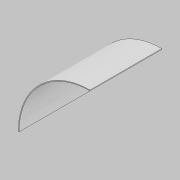
# Autodesk Inventor part: cover2_shell_large
Saved by Autodesk Inventor 2021 (Build 250183000, 183)
## iProperties
Created: 2021-05-31
Part Number: cover2_shell_large
Material: Generic
Document SubType Name: Modeling
Designer: Watchdog
Density: 1 g/cm^3
Appearance: Default
Author: Watchdog
Autodesk Inventor part; units mm, degrees
ref_plane "YZ Plane" through (0, 0, 0) normal (1, 0, 0) x (0, 1, 0)
ref_plane "XZ Plane" through (0, 0, 0) normal (0, 1, 0) x (-1, 0, 0)
ref_plane "XY Plane" through (0, 0, 0) normal (0, 0, 1) x (1, 0, 0)
sketch "Sketch1" plane through (0, 0, 0) normal (0, 0, 1) x (1, 0, 0)
  arc A0 (0, 900) -> (-900, 0) centre (0, 0) ccw
  arc A1 (0, 890) -> (-890, 0) centre (0, 0) ccw
  line L0 (-900, 0) -> (-890, 0)
  line L1 (0, 900) -> (0, 890)
  dimension "d0" = 10
  dimension "d1" = 900
  dimension "d2" = 0
  dimension "d3" = 0
  constraints: 4 end point, 4 point on circle, 2 centre point, 1 coincident, 1 horizontal, 1 perpendicular
  measures "d0" radial gap between concentric circles of A0 A1
  measures "d1" radius of A0
  measures "d2" distance from line of point (0, 0) L0
  measures "d3" distance from line of point (0, 0) L1
extrude "Extrusion1" add sketch "Sketch1" along normal blind 900
equation "\"d1\" = cover_height_main"
equation "\"d4\" = cover_mountHole_xSpacing"
equation "\"cover_height_main\" = 900"
equation "\"cover_mountHole_xSpacing\" = 900"
equation "\"hoop_angle_z\" = 45deg"
equation "\"hoop_bearing_length\" = 5deg"
equation "\"hoop_cable_diam\" = 5"
equation "\"hoop_cable_pulley_diam\" = 22"
equation "\"rack_tooth_addendum\" = 5"
equation "\"rack_tooth_dedendum\" = 5"
equation "\"rack_tooth_thickness\" = 5"
equation "\"secure_arm_angle\" = 20deg"
equation "\"secure_arm_hold_length\" = 35"
equation "\"secure_arm_radii\" = 9"
equation "\"support_baseClamp_platformLengthBuffer\" = 35"
equation "\"support_baseClamp_platformThickness\" = 15"
equation "\"support_baseClamp_platformWidthBuffer\" = 0"
equation "\"support_baseClamp_sleeveHoleDiameter\" = 12"
equation "\"support_baseClamp_sleeveSweepTerminationAngle\" = 55deg"
equation "\"support_baseClamp_thickness\" = 8"
equation "\"support_frame_endHoleBuffer\" = 25"
equation "\"support_frame_squareBarFillet\" = 2"
equation "\"support_frame_squareBarThickness\" = 5"
equation "\"hoop_tabs_thickness\" = 6"
equation "\"hoop_tabs_hole\" = 4"
equation "\"wheelchair_deployed_width\" = 635"
equation "\"wheelchair_deployed_length\" = 1067"
equation "\"wheelchair_deployed_height\" = 914"
body "Solid1"
